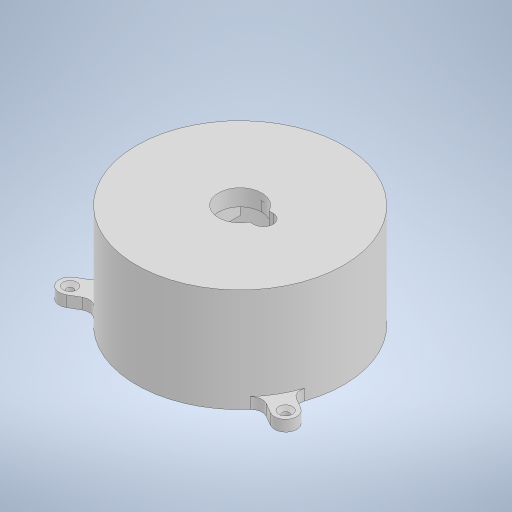
# Autodesk Inventor part: base
Saved by Autodesk Inventor 2023 (Build 270158000, 158)
## iProperties
Created: 2023-04-29
Part Number: base
Material: 一般
Document SubType Name: Modeling
Designer: taka2
Density: 1 g/cm^3
Appearance: 既定
Author: taka2
Autodesk Inventor part; units mm, degrees
ref_plane "XZ Plane" through (0, 0, 0) normal (0, 1, 0) x (-1, 0, 0)
ref_plane "XY Plane" through (0, 0, 0) normal (0, 0, 1) x (1, 0, 0)
sketch "スケッチ1" plane through (0, 0, 0) normal (0, 1, 0) x (-1, 0, 0)
  circle A0 centre (0, 0) radius 30
  circle A1 centre (0, 0) radius 28
  line L0 (-17.5, -7.5) -> (17.5, -7.5)
  line L1 (17.5, -7.5) -> (17.5, 7.5)
  line L2 (17.5, 7.5) -> (-17.5, 7.5)
  line L3 (-17.5, 7.5) -> (-17.5, -7.5)
  line L4 (97.1207, 0) -> (-153.0696, 0)
  line L5 (0, -103.0521) -> (0, 127.3799)
  line L6 (3.2, -29.8288) -> (3.2, -36)
  arc A2 (-3.2, -36) -> (3.2, -36) centre (0, -36) ccw
  line L7 (-3.2, -36) -> (-3.2, -29.8288)
  circle A3 centre (0, -36) radius 1
  arc A4 (32.7769, 15.2287) -> (29.5769, 20.7713) centre (31.1769, 18) ccw
  circle A5 centre (31.1769, 18) radius 1
  line L8 (32.7769, 15.2287) -> (27.4325, 12.1431)
  line L9 (24.2325, 17.6857) -> (29.5769, 20.7713)
  arc A6 (-29.5769, 20.7713) -> (-32.7769, 15.2287) centre (-31.1769, 18) ccw
  circle A7 centre (-31.1769, 18) radius 1
  line L10 (-29.5769, 20.7713) -> (-24.2325, 17.6857)
  line L11 (-27.4325, 12.1431) -> (-32.7769, 15.2287)
  dimension "d0" = 35
  dimension "d1" = 15
  dimension "d2" = 56
  dimension "d3" = 2
  dimension "d4" = 3.2
  dimension "d5" = 36
  dimension "d6" = 2
  dimension "d9" = 360
  constraints: 24 end point, 8 centre point, 8 point on circle, 5 coincident, 3 point on line, 3 vertical, 2 horizontal, 2 parallel, 1 perpendicular, 1 tangent, 34 other
  measures "d0" distance of L1.end L2.end
  measures "d1" distance of L0.end L1.end
  measures "d2" diameter of A1
  measures "d3" radial gap between concentric circles of A0 A1
  measures "d4" radius of A2
  measures "d5" distance of A0.centre A2.centre
  measures "d6" diameter of A3
extrude "押し出し1" add sketch "スケッチ1" along normal blind 28 contours L4 A1 L5 A0 | A0 L5 A1 L4 | A0 L4 A1 L5 | A1 L4 A0 L5
extrude "押し出し2" add sketch "スケッチ1" along normal blind 3.2 contours A0 L9 A4 L8 | L6 A2 L5 A3 A0 | L5 A3 A2 L7 A0 | A0 L11 A6 L10
sketch "スケッチ2" plane through (0, 28, 0) normal (0, 1, 0) x (1, 0, 0)
  circle A0 centre (0, 0) radius 30
  circle A1 centre (0, 0) radius 30 projected
  constraints: 1 centre point, 1 coincident, 1 concentric
extrude "押し出し3" add sketch "スケッチ2" along normal blind 2
sketch "スケッチ3" plane through (0, 28, 0) normal (0, -1, 0) x (1, 0, 0)
  line L0 (-10.75, -6.25) -> (21.25, -6.25)
  line L1 (21.25, -6.25) -> (21.25, 6.25)
  line L2 (21.25, 6.25) -> (-10.75, 6.25)
  line L3 (-10.75, 6.25) -> (-10.75, -6.25)
  line L4 (-52.7206, 0) -> (77.3772, 0) construction
  line L5 (0, 47.1232) -> (0, -27.9509)
  line L6 (-6.25, 6.25) -> (-6.25, -6.25)
  line L7 (16.75, 6.25) -> (16.75, -6.25)
  arc A0 (5.5877, 2.8) -> (5.5877, -2.8) centre (0, 0) ccw
  line L8 (6.75, 2.8) -> (5.5877, 2.8)
  line L9 (6.75, -2.8) -> (5.5877, -2.8)
  circle A1 centre (-8.5, 0) radius 1
  circle A2 centre (19, 0) radius 1
  arc A3 (6.75, -2.8) -> (6.75, 2.8) centre (6.75, 0) ccw
  point P0 (0, -6.25)
  point P1 (0, 6.25)
  point P2 (-6.25, 0)
  dimension "d17" = 4.5
  dimension "d18" = 4.5
  dimension "d19" = 2
  dimension "d20" = 2.25
  dimension "d21" = 2.25
  dimension "d22" = 13
  dimension "d23" = 12.5
  dimension "d24" = 23
  dimension "d26" = 2.8
  constraints: 20 end point, 9 point on line, 4 centre point, 4 parallel, 4 point on circle, 4 tangent, 3 perpendicular, 2 horizontal, 1 equal radius, 1 vertical, 1 other
  measures "d17" distance of L6.end L0.start
  measures "d18" distance of L0.end L7.end
  measures "d19" diameter of A2
  measures "d20" distance from line of L1 A2.centre
  measures "d21" distance from line of L3 A1.centre
  measures "d22" distance from line of A3.centre L6
  measures "d23" distance of L0.end L1.end
  measures "d24" distance of L7.end L6.end
  measures "d26" radius of A3
extrude "押し出し4" cut sketch "スケッチ3" against normal through all contours A0 L5 | L5 A0 L8 A3 L9
extrude "押し出し5" add sketch "スケッチ3" along normal blind 2.8 contours L6 A0 L0 | A0 L9 A3 L8 L2 L7 L0 | L6 L2 A0
extrude "押し出し6" add sketch "スケッチ3" along normal blind 6.8 contours L3 L2 L6 L0 | L7 L2 L1 L0
ref_plane "作業平面1" through (-30, 0, 0) normal (1, 0, 0) x (0, 1, 0)
sketch "スケッチ4" plane through (-30, 0, 0) normal (1, 0, 0) x (0, 1, 0)
  line L0 (-6.8871, 0) -> (24.1455, 0)
  line L1 (0, -3) -> (1.8, -3)
  line L2 (2.8, -2) -> (2.8, 2)
  line L3 (1.8, 3) -> (0, 3)
  line L4 (0, 3) -> (0, -3)
  arc A0 (1.8, -3) -> (2.8, -2) centre (1.8, -2) ccw
  arc A1 (2.8, 2) -> (1.8, 3) centre (1.8, 2) ccw
  point P0 (0, 0)
  point P1 (2.8, 3)
  point P2 (2.8, -3)
  dimension "d34" = 6
  dimension "d35" = 2.8
  dimension "d36" = 1
  dimension "d37" = 1
  constraints: 10 end point, 5 point on line, 4 point on circle, 4 tangent, 2 centre point, 2 horizontal, 2 parallel, 1 midpoint, 1 perpendicular, 1 other
  measures "d34" distance of point (2.8, -3) point (2.8, 3)
  measures "d35" distance of point (2.8, 3) L3.end
  measures "d36" radius of A0
  measures "d37" radius of A1
extrude "押し出し7" cut sketch "スケッチ4" along normal up to surface
fillet "フィレット1" radius 3.2 6 edges at (24.2325, 1.6, 17.6857) (27.4325, 1.6, 12.1431) (3.2, 1.6, -29.8288) (-3.2, 1.6, -29.8288) (-27.4325, 1.6, 12.1431) (-24.2325, 1.6, 17.6857)
sketch "スケッチ5" plane through (0, 3.2, 0) normal (0, 1, 0) x (1, 0, 0)
  circle A0 centre (31.1769, -18) radius 1 projected
  circle A1 centre (-31.1769, -18) radius 1 projected
  circle A2 centre (0, 36) radius 1 projected
  point P0 (0, 0)
  constraints: 3 coincident
hole "穴1" at (31.1769, 3.2, 18) at (-31.1769, 3.2, 18) at (0, 3.2, -36) direction (0, -1, 0) diameter 2 end through all countersink diameter 4 countersink angle 90
